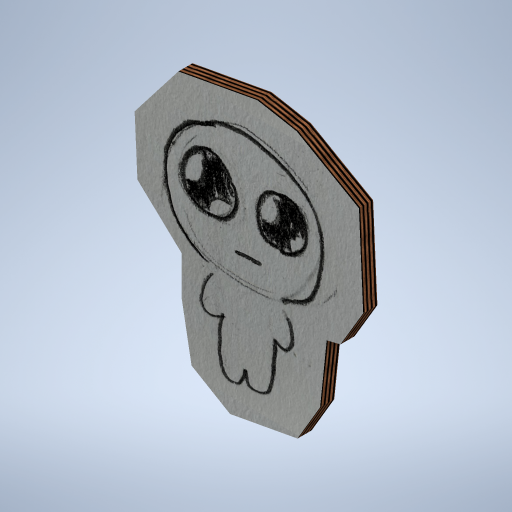
# Autodesk Inventor part: tbh
Saved by Autodesk Inventor 2023 (Build 270158000, 158)
## iProperties
Created: 2024-07-02
Part Number: tbh
Material: Generic
Document SubType Name: Modeling
Designer: Student-27
Density: 1 g/cm^3
Appearance: Default
Author: Student-27
Autodesk Inventor part; units mm, degrees
ref_plane "YZ Plane" through (0, 0, 0) normal (1, 0, 0) x (0, 1, 0)
ref_plane "XZ Plane" through (0, 0, 0) normal (0, 1, 0) x (-1, 0, 0)
ref_plane "XY Plane" through (0, 0, 0) normal (0, 0, 1) x (1, 0, 0)
sketch "Sketch1" plane through (0, 0, 0) normal (0, 0, 1) x (1, 0, 0)
  line L0 (291.1774, -13.0799) -> (402.8839, -76.8892)
  line L1 (402.8839, -76.8892) -> (410.5344, -236.5925)
  line L2 (410.5344, -236.5925) -> (369.664, -305.2907)
  line L3 (369.664, -305.2907) -> (345.0261, -311.3937)
  line L4 (345.0261, -311.3937) -> (333.128, -421.456)
  line L5 (333.128, -421.456) -> (292.5108, -490.3287)
  line L6 (292.5108, -490.3287) -> (171.3005, -512.6841)
  line L7 (171.3005, -512.6841) -> (102.1926, -471.9281)
  line L8 (102.1926, -471.9281) -> (84.4874, -375.9311)
  line L9 (84.4874, -375.9311) -> (84.4874, -306.0658)
  line L10 (84.4874, -306.0658) -> (4.9697, -231.3611)
  line L11 (4.9697, -231.3611) -> (0, -127.6185)
  line L12 (0, -127.6185) -> (78.5872, -26.1598)
  line L13 (78.5872, -26.1598) -> (220.4253, 0)
  line L14 (220.4253, 0) -> (291.1774, -13.0799)
  line L15 (0, 0) -> (409.1185, 0)
  line L16 (409.1185, 0) -> (409.1185, -512.6841)
  line L17 (409.1185, -512.6841) -> (0, -512.6841)
  line L18 (0, -512.6841) -> (0, 0)
  point P0 (0, 0)
  dimension "d11" = 409.1185
  dimension "d14" = 512.6841
  constraints: 38 end point, 4 perpendicular, 3 parallel, 1 horizontal, 1 point on line, 1 vertical
  measures "d11" distance of L15.start L15.end
  measures "d14" distance of L17.end L15.start
extrude "Extrusion1" add sketch "Sketch1" against normal blind 25.4 contours L0 L1 L16 L2 L3 L4 L5 L6 L7 L8 L9 L10 L11 L12 L13 L14 | L1 L2 L16
body "Solid1"
